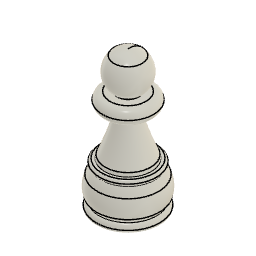
Pawn (Autodesk Fusion 360 design; units mm, degrees)
Autodesk Fusion 360 part; units mm, degrees
sketch "Pawn" plane through (0, 0, 0) normal (1, 0, 0) x (0, 1, 0)
  line L0 (-8.5328, 13.1623) -> (8.8695, 13.1623)
  spline S0 degree 3 poles (8.8695, 13.1623) (9.2816, 13.335) (9.5806, 13.6432) (9.4727, 14.1724) knots 0 0 0 0 1 1 1 1
  spline S1 degree 3 poles (9.4727, 14.1724) (9.3643, 14.7055) (9.0964, 14.9423) (8.7537, 15.0508) knots 0 0 0 0 1 1 1 1
  line L1 (8.7537, 15.0508) -> (-8.296, 15.0508)
  spline S2 degree 3 poles (-8.296, 15.0508) (-8.7101, 14.8722) (-8.9231, 14.4866) (-8.935, 13.919) knots 0 0 0 0 1 1 1 1
  spline S3 degree 3 poles (-8.935, 13.919) (-8.9442, 13.4805) (-8.7809, 13.2662) (-8.5328, 13.1623) knots 0 0 0 0 1 1 1 1
  line L2 (-9.146, 2.6961) -> (9.4648, 2.6961)
  spline S4 degree 3 poles (9.4648, 2.6961) (9.9702, 2.9871) (10.2202, 3.5791) (10.4649, 4.1923) knots 0 0 0 0 1 1 1 1
  spline S5 degree 3 poles (10.4649, 4.1923) (11.266, 6.1912) (11.0027, 8.1531) (10.2169, 10.0667) knots 0 0 0 0 1 1 1 1
  spline S6 degree 3 poles (10.2169, 10.0667) (9.816, 11.043) (9.4053, 12.0398) (8.6036, 12.7866) knots 0 0 0 0 1 1 1 1
  line L3 (8.6036, 12.7866) -> (-8.3066, 12.7866)
  spline S7 degree 3 poles (-8.3066, 12.7866) (-8.3655, 12.7529) (-8.4204, 12.7086) (-8.4693, 12.6437) knots 0 0 0 0 1 1 1 1
  spline S8 degree 3 poles (-8.4693, 12.6437) (-10.3161, 10.1858) (-11.5034, 7.571) (-10.3737, 4.4231) knots 0 0 0 0 1 1 1 1
  spline S9 degree 3 poles (-10.3737, 4.4231) (-9.9794, 3.3245) (-9.7479, 2.874) (-9.146, 2.6961) knots 0 0 0 0 1 1 1 1
  line L4 (9.5144, 2.321) -> (-9.4992, 2.321)
  spline S10 degree 3 poles (-9.4992, 2.321) (-10.1871, 2.0975) (-10.5847, 1.4109) (-10.5033, 0.5496) knots 0 0 0 0 1 1 1 1
  spline S11 degree 3 poles (-10.5033, 0.5496) (-10.412, -0.4187) (-9.6255, 0.0264) (-9.1996, 0.0211) knots 0 0 0 0 1 1 1 1
  spline S12 degree 3 poles (-9.1996, 0.0211) (-5.375, -0.0232) (-1.5498, 0) (2.2748, 0.0039) knots 0 0 0 0 1 1 1 1
  spline S13 degree 3 poles (2.2748, 0.0039) (4.8392, 0.0053) (7.405, 0.0258) (9.9695, 0.0039) knots 0 0 0 0 1 1 1 1
  spline S14 degree 3 poles (9.9695, 0.0039) (10.6085, -0.0027) (10.7441, 0.2156) (10.6138, 0.8103) knots 0 0 0 0 1 1 1 1
  spline S15 degree 3 poles (10.6138, 0.8103) (10.4279, 1.6629) (10.1693, 2.0889) (9.5144, 2.321) knots 0 0 0 0 1 1 1 1
  spline S16 degree 3 poles (3.5044, 28.788) (3.3476, 29.458) (3.3218, 29.759) (3.5613, 29.8926) knots 0 0 0 0 1 1 1 1
  line L5 (3.5613, 29.8926) -> (6.0113, 29.8926)
  spline S17 degree 3 poles (6.0113, 29.8926) (7.4057, 29.8926) (8.5361, 31.023) (8.5361, 32.418) knots 0 0 0 0 1 1 1 1
  spline S18 degree 3 poles (8.5361, 32.418) (8.5361, 33.8124) (7.4057, 34.9435) (6.0113, 34.9435) knots 0 0 0 0 1 1 1 1
  line L6 (6.0113, 34.9435) -> (3.4687, 34.9435)
  spline S19 degree 3 poles (3.4687, 34.9435) (3.4449, 34.9514) (3.4217, 34.958) (3.3986, 34.9666) knots 0 0 0 0 1 1 1 1
  spline S20 degree 3 poles (3.3986, 34.9666) (7.5611, 37.9399) (7.1166, 42.7136) (4.7056, 45.2841) knots 0 0 0 0 1 1 1 1
  spline S21 degree 3 poles (4.7056, 45.2841) (2.3779, 47.7652) (-2.0036, 48.0404) (-4.6659, 45.2424) knots 0 0 0 0 1 1 1 1
  spline S22 degree 3 poles (-4.6659, 45.2424) (-6.7502, 43.0523) (-7.7272, 38.4313) (-3.3225, 34.9435) knots 0 0 0 0 1 1 1 1
  line L7 (-3.3225, 34.9435) -> (-6.0107, 34.9435)
  spline S23 degree 3 poles (-6.0107, 34.9435) (-7.405, 34.9435) (-8.5361, 33.8124) (-8.5361, 32.418) knots 0 0 0 0 1 1 1 1
  spline S24 degree 3 poles (-8.5361, 32.418) (-8.5361, 31.023) (-7.405, 29.8926) (-6.0107, 29.8926) knots 0 0 0 0 1 1 1 1
  line L8 (-6.0107, 29.8926) -> (-3.6327, 29.8926)
  spline S25 degree 3 poles (-3.6327, 29.8926) (-3.1571, 29.7352) (-3.2306, 29.3204) (-3.5104, 28.2184) knots 0 0 0 0 1 1 1 1
  spline S26 degree 3 poles (-3.5104, 28.2184) (-4.5436, 24.1419) (-5.6131, 20.0759) (-7.2172, 16.1786) knots 0 0 0 0 1 1 1 1
  spline S27 degree 3 poles (-7.2172, 16.1786) (-7.3739, 15.7989) (-7.3395, 15.6322) (-7.1702, 15.5423) knots 0 0 0 0 1 1 1 1
  line L9 (-7.1702, 15.5423) -> (7.741, 15.5423)
  spline S28 degree 3 poles (7.741, 15.5423) (7.9931, 15.7288) (7.8773, 15.9689) (7.581, 16.6588) knots 0 0 0 0 1 1 1 1
  spline S29 degree 3 poles (7.581, 16.6588) (5.8896, 20.5905) (4.4847, 24.6188) (3.5044, 28.788) knots 0 0 0 0 1 1 1 1
  line L10 (0, 47.2438) -> (0, 0)
  constraint coincident S21 L10.start
  constraint coincident S12 L10.end
  constraint perpendicular L2 L10
revolve "Revolve1" add sketch "Pawn" angle 360 about axis through (0, 0, 47.2438) along (0, 0, -1) contours L0 S0 S1 L1 L10 | L2 S4 S5 S6 L3 L10 | L4 S12 S13 S14 S15 L10 | S16 L5 S17 S18 L6 S19 S20 S21 L9 S28 S29 L10 makes body 1 at (-0.4836, 4.5243, 13.1623) makes body 2 at (6.0409, -8.8604, 8.5257) makes body 3 at (-0.8928, 5.9233, 20.6243) makes body 4 at (-0.3691, 7.3955, 0.0139)
move_body "Align1" bodies 2 to x (1, 0, 0) y (0, 1, 0) z (0, 0, 1) at (0, 0, -0.375)
move_body "Align2" bodies 1 to x (1, 0, 0) y (0, 1, 0) z (0, 0, 1) at (0, 0, -0.7508)
move_body "Align3" bodies 3 to x (1, 0, 0) y (0, 1, 0) z (0, 0, 1) at (0, 0, -1.2422)
combine "Combine1" operation add target body 4 tool bodies 2 1 3
named bodies: "Pawn"
